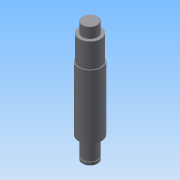
# Autodesk Inventor part: 齿轮150配件
Saved by Autodesk Inventor 2015 (Build 190159000, 159)
## iProperties
Created: 2017-05-27
Part Number: 齿轮150配件
Material: 常规
Document SubType Name: Modeling
Designer: Administrator
Density: 1 g/cm^3
Appearance: 默认
Author: Administrator
Autodesk Inventor part; units mm, degrees
ref_plane "YZ Plane" through (0, 0, 0) normal (1, 0, 0) x (0, 1, 0)
ref_plane "XY Plane" through (0, 0, 0) normal (0, 0, 1) x (1, 0, 0)
sketch "草图1" plane through (0, 0, 0) normal (0, 0, 1) x (1, 0, 0)
  circle A0 centre (0, 0) radius 10
  dimension "d0" = 20
  constraints: 1 centre point, 1 coincident
  measures "d0" diameter of A0
extrude "拉伸1" add sketch "草图1" along normal blind 28.378
sketch "草图2" plane through (0, 0, 28.378) normal (0, 0, 1) x (1, 0, 0)
  circle A0 centre (0, 0) radius 15
  dimension "d3" = 30
  constraints: 1 centre point, 1 coincident
  measures "d3" diameter of A0
extrude "拉伸2" add sketch "草图2" along normal blind 83.422
sketch "草图3" plane through (0, 0, 111.8) normal (0, 0, 1) x (1, 0, 0)
  circle A0 centre (0, 0) radius 14
  dimension "d6" = 28
  constraints: 1 centre point, 1 coincident
  measures "d6" diameter of A0
extrude "拉伸3" add sketch "草图3" along normal blind 32
sketch "草图4" plane through (0, 0, 143.8) normal (0, 0, 1) x (1, 0, 0)
  circle A0 centre (0, 0) radius 10
  dimension "d9" = 20
  constraints: 1 centre point, 1 coincident
  measures "d9" diameter of A0
extrude "拉伸4" add sketch "草图4" along normal blind 14
ref_plane "工作平面1" through (0, 10, 0) normal (0, 1, 0) x (-1, 0, 0)
sketch "草图5" plane through (0, 10, 0) normal (0, 1, 0) x (-1, 0, 0)
  line L0 (-3, 22.789) -> (3, 22.789)
  line L1 (3, 22.789) -> (3, 10.789)
  line L2 (3, 10.789) -> (-3, 10.789)
  line L3 (-3, 10.789) -> (-3, 22.789)
  arc A0 (3, 22.789) -> (-3, 22.789) centre (0, 22.789) ccw
  arc A1 (-3, 10.789) -> (3, 10.789) centre (0, 10.789) ccw
  line L4 (0, 0) -> (0, -4.7288)
  line L5 (10, 28.378) -> (-10, 28.378) projected
  dimension "d12" = 4.7288
  dimension "d13" = 6
  dimension "d14" = 12
  dimension "d21" = 5.589
  constraints: 10 end point, 4 point on circle, 4 tangent, 2 centre point, 2 parallel, 1 horizontal, 1 midpoint, 1 perpendicular, 1 point on line, 1 vertical
  measures "d12" distance of L4.start L4.end
  measures "d13" distance of L0.start L0.end
  measures "d14" distance of L0.end L1.end
  measures "d21" distance between parallel lines of L5 L0
extrude "拉伸5" cut sketch "草图5" against normal blind 2.5
chamfer "倒角1" distance 0.5 angle 45 2 edges at (-10, 0, 0) (-10, 0, 157.8)
sketch "草图6" plane through (0, 0, 0) normal (0, 1, 0) x (-1, 0, 0)
  line L0 (14.4109, 5.2) -> (9.175, 5.2)
  line L1 (9.175, 5.2) -> (9.175, 4)
  line L2 (9.175, 4) -> (14.4109, 4)
  line L3 (14.4109, 4) -> (14.4109, 5.2)
  line L4 (9.5, 0) -> (-9.5, 0) projected
  line L5 (0, 0) -> (0, -3.7924)
  dimension "d22" = 4
  dimension "d23" = 1.2
  dimension "d24" = 3.7924
  dimension "d25" = 9.175
  dimension "d26" = 5.2359
  constraints: 10 end point, 2 parallel, 1 horizontal, 1 perpendicular, 1 vertical
  measures "d22" distance between parallel lines of L4 L2
  measures "d23" distance of L2.end L0.start
  measures "d24" distance of L5.start L5.end
  measures "d25" distance between parallel lines of L5 L1
  measures "d26" distance of L1.end L2.end
revolve "旋转1" cut sketch "草图6" angle 360 about axis through (0, 0, 0) along (0, 0, -1)
